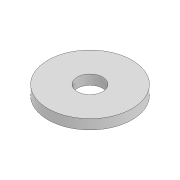
# Autodesk Inventor part: Horizontal_bar_spacer_small_template
Saved by Autodesk Inventor 2022 (Build 260153000, 153)
## iProperties
Created: 2022-09-09
Part Number: Horizontal_bar_spacer_small_template
Material: Generic
Document SubType Name: Modeling
Designer: dell
Density: 1 g/cm^3
Appearance: Default
Mass: 0.124054 g
Surface Area: 1.76856 cm^2
Volume: 0.124054 cm^3
Author: dell
Autodesk Inventor part; units mm, degrees
ref_plane "YZ Plane" through (0, 0, 0) normal (1, 0, 0) x (0, 1, 0)
ref_plane "XZ Plane" through (0, 0, 0) normal (0, 1, 0) x (-1, 0, 0)
ref_plane "XY Plane" through (0, 0, 0) normal (0, 0, 1) x (1, 0, 0)
sketch "Sketch1" plane through (0, 0, 0) normal (0, 1, 0) x (-1, 0, 0)
  circle A0 centre (0, 0) radius 1.55
  circle A1 centre (0, 0) radius 5
  circle A2 centre (0, 0) radius 5.2
  circle A3 centre (0, 0) radius 17.2
  dimension "d0" = 3.1
  dimension "d1" = 10
  dimension "d4" = 0.2
  dimension "d5" = 12
  constraints: 4 centre point, 2 coincident
  measures "d0" diameter of A0
  measures "d1" diameter of A1
  measures "d4" radial gap between concentric circles of A1 A2
  measures "d5" radial gap between concentric circles of A2 A3
extrude "Extrusion1" add sketch "Sketch1" along normal blind 4 contours A3
body "Solid1"
